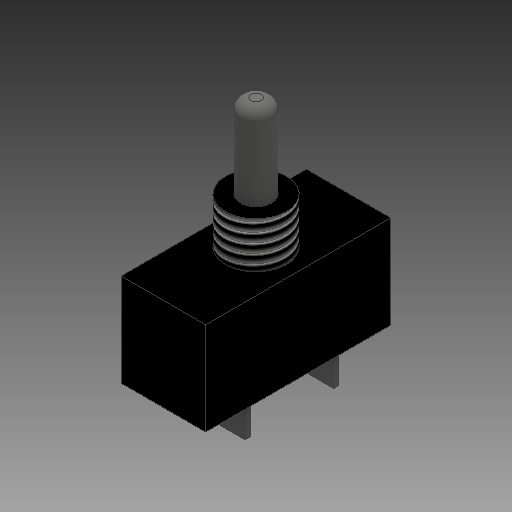
# Autodesk Inventor part: Schalter
Saved by Autodesk Inventor 2019 (Build 230136000, 136)
## iProperties
Created: 2018-05-16
Part Number: Schalter
Material: Generic
Document SubType Name: Modeling
Designer: Phil Erle
Density: 1 g/cm^3
Appearance: Default
Author: Phil Erle
Autodesk Inventor part; units mm, degrees
ref_plane "YZ Plane" through (0, 0, 0) normal (1, 0, 0) x (0, 1, 0)
ref_plane "XZ Plane" through (0, 0, 0) normal (0, 1, 0) x (-1, 0, 0)
ref_plane "XY Plane" through (0, 0, 0) normal (0, 0, 1) x (1, 0, 0)
sketch "Sketch1" plane through (0, 0, 0) normal (0, 0, 1) x (1, 0, 0)
  line L0 (-8.1, -17.75) -> (8.1, -17.75)
  line L1 (8.1, -17.75) -> (8.1, 17.75)
  line L2 (8.1, 17.75) -> (-8.1, 17.75)
  line L3 (-8.1, 17.75) -> (-8.1, -17.75)
  line L4 (-8.1, -17.75) -> (8.1, 17.75) construction
  line L5 (8.1, -17.75) -> (-8.1, 17.75) construction
  point P0 (0, 0)
  dimension "d0" = 16.2
  dimension "d1" = 35.5
  constraints: 12 end point, 2 midpoint, 2 parallel, 1 horizontal, 1 perpendicular
  measures "d0" distance of L1.end L2.end
  measures "d1" distance of L0.end L1.end
extrude "Extrusion1" add sketch "Sketch1" along normal blind 17.8
sketch "Sketch2" plane through (0, 0, 17.8) normal (0, 0, 1) x (1, 0, 0)
  circle A0 centre (0, 0) radius 5.85
  dimension "d4" = 11.7
  constraints: 1 centre point, 1 coincident
  measures "d4" diameter of A0
extrude "Extrusion2" add sketch "Sketch2" along normal blind 8.8
sketch "Sketch3" plane through (0, 0, 26.6) normal (0, 0, 1) x (1, 0, 0)
  circle A0 centre (0, 0) radius 3
  dimension "d7" = 6
  constraints: 1 centre point, 1 coincident
  measures "d7" diameter of A0
extrude "Extrusion3" add sketch "Sketch3" along normal blind 16
fillet "Fillet1" radius 2 1 edges at (-3, 0, 42.6)
sketch "Sketch4" plane through (0, 0, 0) normal (0, 0, -1) x (-1, 0, 0)
  line L0 (-3.15, 12.75) -> (3.15, 12.75)
  line L1 (3.15, 12.75) -> (3.15, 11.75)
  line L2 (3.15, 11.75) -> (-3.15, 11.75)
  line L3 (-3.15, 11.75) -> (-3.15, 12.75)
  line L4 (-3.15, 12.75) -> (3.15, 11.75) construction
  line L5 (3.15, 12.75) -> (-3.15, 11.75) construction
  line L6 (-3.15, -4.25) -> (3.15, -4.25)
  line L7 (3.15, -4.25) -> (3.15, -5.25)
  line L8 (3.15, -5.25) -> (-3.15, -5.25)
  line L9 (-3.15, -5.25) -> (-3.15, -4.25)
  line L10 (-3.15, -4.25) -> (3.15, -5.25) construction
  line L11 (3.15, -4.25) -> (-3.15, -5.25) construction
  line L12 (-8.1, 17.75) -> (8.1, 17.75) projected
  line L13 (8.1, -17.75) -> (-8.1, -17.75) projected
  point P0 (0, 0)
  point P1 (0, 12.25)
  point P2 (0, -4.75)
  point P3 (0, 12.25)
  point P4 (0, -4.75)
  dimension "d11" = 6.3
  dimension "d12" = 1
  dimension "d13" = 6.3
  dimension "d14" = 1
  dimension "d15" = 5
  dimension "d16" = 12.5
  constraints: 24 end point, 6 midpoint, 4 parallel, 2 horizontal, 2 perpendicular, 2 vertical alignment
  measures "d11" distance of L1.end L2.end
  measures "d12" distance of L0.end L1.end
  measures "d13" distance of L7.end L8.end
  measures "d14" distance of L6.end L7.end
  measures "d15" distance between parallel lines of L12 L0
  measures "d16" distance between parallel lines of L13 L8
extrude "Extrusion4" add sketch "Sketch4" along normal blind 10
thread "Thread1" size "M12x1.75" class "6g" standard "ANSI Metric M Profile" full length
body "Solid1"
